Autodesk Fusion 360 part; units mm, degrees
(part 5 of 6)
sketch "b left  projection" plane through (0, 0, 0) normal (0, 0, 1) x (1, 0, 0) in component "b left component"
  arc A0 (116.825, 236.4194) -> (116.825, 235.2313) centre (117.6356, 235.8254) ccw
  arc A1 (118.4308, 236.44) -> (116.8405, 236.44) centre (117.6356, 235.8254) ccw
  arc A2 (105.08, 252.4508) -> (105.08, 250.8605) centre (105.6946, 251.6556) ccw
  arc A3 (116.8405, 226.6) -> (118.4308, 226.6) centre (117.6356, 227.2146) ccw
  arc A4 (93.7113, 250.845) -> (94.8994, 250.845) centre (94.3054, 251.6556) ccw
  arc A5 (116.825, 216.4194) -> (116.825, 215.2313) centre (117.6356, 215.8254) ccw
  arc A6 (85.08, 252.4508) -> (85.08, 250.8605) centre (85.6946, 251.6556) ccw
  arc A7 (116.8405, 206.6) -> (118.4308, 206.6) centre (117.6356, 207.2146) ccw
  arc A8 (73.7113, 250.845) -> (74.8994, 250.845) centre (74.3054, 251.6556) ccw
  arc A9 (105.08, 192.1795) -> (105.08, 190.5892) centre (105.6946, 191.3844) ccw
  arc A10 (65.08, 252.4508) -> (65.08, 250.8605) centre (65.6946, 251.6556) ccw
  arc A11 (94.8994, 192.195) -> (93.7113, 192.195) centre (94.3054, 191.3844) ccw
  arc A12 (53.7113, 250.845) -> (54.8994, 250.845) centre (54.3054, 251.6556) ccw
  arc A13 (85.08, 192.1795) -> (85.08, 190.5892) centre (85.6946, 191.3844) ccw
  arc A14 (45.08, 252.4508) -> (45.08, 250.8605) centre (45.6946, 251.6556) ccw
  arc A15 (74.8994, 192.195) -> (73.7113, 192.195) centre (74.3054, 191.3844) ccw
  arc A16 (33.7113, 250.845) -> (34.8994, 250.845) centre (34.3054, 251.6556) ccw
  arc A17 (65.08, 192.1795) -> (65.08, 190.5892) centre (65.6946, 191.3844) ccw
  arc A18 (25.08, 252.4508) -> (25.08, 250.8605) centre (25.6946, 251.6556) ccw
  arc A19 (54.8994, 192.195) -> (53.7113, 192.195) centre (54.3054, 191.3844) ccw
  arc A20 (13.7113, 250.845) -> (14.8994, 250.845) centre (14.3054, 251.6556) ccw
  arc A21 (45.08, 192.1795) -> (45.08, 190.5892) centre (45.6946, 191.3844) ccw
  arc A22 (3.175, 235.2313) -> (3.175, 236.4194) centre (2.3644, 235.8254) ccw
  arc A23 (34.8994, 192.195) -> (33.7113, 192.195) centre (34.3054, 191.3844) ccw
  arc A24 (1.5692, 226.6) -> (3.1595, 226.6) centre (2.3644, 227.2146) ccw
  arc A25 (25.08, 192.1795) -> (25.08, 190.5892) centre (25.6946, 191.3844) ccw
  arc A26 (3.175, 215.2313) -> (3.175, 216.4194) centre (2.3644, 215.8254) ccw
  arc A27 (1.5692, 206.6) -> (3.1595, 206.6) centre (2.3644, 207.2146) ccw
  arc A28 (14.8994, 192.195) -> (13.7113, 192.195) centre (14.3054, 191.3844) ccw
  arc A29 (66.2887, 192.195) -> (65.1006, 192.195) centre (65.6946, 191.3844) ccw
  arc A30 (94.92, 250.8605) -> (94.92, 252.4508) centre (94.3054, 251.6556) ccw
  arc A31 (105.1006, 250.845) -> (106.2887, 250.845) centre (105.6946, 251.6556) ccw
  arc A32 (3.175, 206.6206) -> (3.175, 207.8087) centre (2.3644, 207.2146) ccw
  arc A33 (3.1595, 216.44) -> (1.5692, 216.44) centre (2.3644, 215.8254) ccw
  arc A34 (3.175, 226.6206) -> (3.175, 227.8087) centre (2.3644, 227.2146) ccw
  arc A35 (3.1595, 236.44) -> (1.5692, 236.44) centre (2.3644, 235.8254) ccw
  arc A36 (118.4308, 216.44) -> (116.8405, 216.44) centre (117.6356, 215.8254) ccw
  arc A37 (54.92, 190.5892) -> (54.92, 192.1795) centre (54.3054, 191.3844) ccw
  arc A38 (86.2887, 192.195) -> (85.1006, 192.195) centre (85.6946, 191.3844) ccw
  arc A39 (74.92, 190.5892) -> (74.92, 192.1795) centre (74.3054, 191.3844) ccw
  arc A40 (106.2887, 192.195) -> (105.1006, 192.195) centre (105.6946, 191.3844) ccw
  arc A41 (54.92, 250.8605) -> (54.92, 252.4508) centre (54.3054, 251.6556) ccw
  arc A42 (65.1006, 250.845) -> (66.2887, 250.845) centre (65.6946, 251.6556) ccw
  arc A43 (85.1006, 250.845) -> (86.2887, 250.845) centre (85.6946, 251.6556) ccw
  arc A44 (14.92, 250.8605) -> (14.92, 252.4508) centre (14.3054, 251.6556) ccw
  arc A45 (14.92, 190.5892) -> (14.92, 192.1795) centre (14.3054, 191.3844) ccw
  arc A46 (34.92, 190.5892) -> (34.92, 192.1795) centre (34.3054, 191.3844) ccw
  arc A47 (25.1006, 250.845) -> (26.2887, 250.845) centre (25.6946, 251.6556) ccw
  arc A48 (116.825, 207.8087) -> (116.825, 206.6206) centre (117.6356, 207.2146) ccw
  arc A49 (46.2887, 192.195) -> (45.1006, 192.195) centre (45.6946, 191.3844) ccw
  arc A50 (34.92, 250.8605) -> (34.92, 252.4508) centre (34.3054, 251.6556) ccw
  arc A51 (94.92, 190.5892) -> (94.92, 192.1795) centre (94.3054, 191.3844) ccw
  arc A52 (26.2887, 192.195) -> (25.1006, 192.195) centre (25.6946, 191.3844) ccw
  arc A53 (116.825, 227.8087) -> (116.825, 226.6206) centre (117.6356, 227.2146) ccw
  arc A54 (74.92, 250.8605) -> (74.92, 252.4508) centre (74.3054, 251.6556) ccw
  arc A55 (45.1006, 250.845) -> (46.2887, 250.845) centre (45.6946, 251.6556) ccw
  line L0 (116.825, 236.44) -> (116.8405, 236.44)
  line L1 (105.08, 250.845) -> (105.1006, 250.845)
  line L2 (106.2887, 250.845) -> (120, 250.845)
  line L3 (116.825, 226.6) -> (116.825, 226.6206)
  line L4 (116.825, 227.8087) -> (116.825, 235.2313)
  line L5 (116.825, 236.4194) -> (116.825, 236.44)
  line L6 (105.08, 254.02) -> (105.08, 252.4508)
  line L7 (105.08, 250.8605) -> (105.08, 250.845)
  line L8 (120, 226.6) -> (118.4308, 226.6)
  line L9 (116.8405, 226.6) -> (116.825, 226.6)
  line L10 (94.92, 250.845) -> (94.92, 250.8605)
  line L11 (94.92, 252.4508) -> (94.92, 254.02)
  line L12 (116.825, 216.44) -> (116.8405, 216.44)
  line L13 (118.4308, 216.44) -> (120, 216.44)
  line L14 (85.08, 250.845) -> (85.1006, 250.845)
  line L15 (86.2887, 250.845) -> (93.7113, 250.845)
  line L16 (94.8994, 250.845) -> (94.92, 250.845)
  line L17 (85.08, 254.02) -> (85.08, 252.4508)
  line L18 (85.08, 250.8605) -> (85.08, 250.845)
  line L19 (116.825, 206.6) -> (116.825, 206.6206)
  line L20 (116.825, 207.8087) -> (116.825, 215.2313)
  line L21 (116.825, 216.4194) -> (116.825, 216.44)
  line L22 (120, 206.6) -> (118.4308, 206.6)
  line L23 (116.8405, 206.6) -> (116.825, 206.6)
  line L24 (74.92, 250.845) -> (74.92, 250.8605)
  line L25 (74.92, 252.4508) -> (74.92, 254.02)
  line L26 (105.08, 192.195) -> (105.1006, 192.195)
  line L27 (106.2887, 192.195) -> (120, 192.195)
  line L28 (65.08, 250.845) -> (65.1006, 250.845)
  line L29 (66.2887, 250.845) -> (73.7113, 250.845)
  line L30 (74.8994, 250.845) -> (74.92, 250.845)
  line L31 (105.08, 189.02) -> (105.08, 190.5892)
  line L32 (105.08, 192.1795) -> (105.08, 192.195)
  line L33 (65.08, 254.02) -> (65.08, 252.4508)
  line L34 (65.08, 250.8605) -> (65.08, 250.845)
  line L35 (94.92, 192.195) -> (94.92, 192.1795)
  line L36 (94.92, 190.5892) -> (94.92, 189.02)
  line L37 (54.92, 250.845) -> (54.92, 250.8605)
  line L38 (54.92, 252.4508) -> (54.92, 254.02)
  line L39 (85.08, 192.195) -> (85.1006, 192.195)
  line L40 (86.2887, 192.195) -> (93.7113, 192.195)
  line L41 (94.8994, 192.195) -> (94.92, 192.195)
  line L42 (45.08, 250.845) -> (45.1006, 250.845)
  line L43 (46.2887, 250.845) -> (53.7113, 250.845)
  line L44 (54.8994, 250.845) -> (54.92, 250.845)
  line L45 (85.08, 189.02) -> (85.08, 190.5892)
  line L46 (85.08, 192.1795) -> (85.08, 192.195)
  line L47 (45.08, 254.02) -> (45.08, 252.4508)
  line L48 (45.08, 250.8605) -> (45.08, 250.845)
  line L49 (74.92, 192.195) -> (74.92, 192.1795)
  line L50 (74.92, 190.5892) -> (74.92, 189.02)
  line L51 (34.92, 250.845) -> (34.92, 250.8605)
  line L52 (34.92, 252.4508) -> (34.92, 254.02)
  line L53 (65.08, 192.195) -> (65.1006, 192.195)
  line L54 (66.2887, 192.195) -> (73.7113, 192.195)
  line L55 (74.8994, 192.195) -> (74.92, 192.195)
  line L56 (25.08, 250.845) -> (25.1006, 250.845)
  line L57 (26.2887, 250.845) -> (33.7113, 250.845)
  line L58 (34.8994, 250.845) -> (34.92, 250.845)
  line L59 (65.08, 189.02) -> (65.08, 190.5892)
  line L60 (65.08, 192.1795) -> (65.08, 192.195)
  line L61 (25.08, 254.02) -> (25.08, 252.4508)
  line L62 (25.08, 250.8605) -> (25.08, 250.845)
  line L63 (54.92, 192.195) -> (54.92, 192.1795)
  line L64 (54.92, 190.5892) -> (54.92, 189.02)
  line L65 (14.92, 250.845) -> (14.92, 250.8605)
  line L66 (14.92, 252.4508) -> (14.92, 254.02)
  line L67 (0, 250.845) -> (13.7113, 250.845)
  line L68 (14.8994, 250.845) -> (14.92, 250.845)
  line L69 (45.08, 192.195) -> (45.1006, 192.195)
  line L70 (46.2887, 192.195) -> (53.7113, 192.195)
  line L71 (54.8994, 192.195) -> (54.92, 192.195)
  line L72 (3.175, 236.44) -> (3.1595, 236.44)
  line L73 (1.5692, 236.44) -> (0, 236.44)
  line L74 (45.08, 189.02) -> (45.08, 190.5892)
  line L75 (45.08, 192.1795) -> (45.08, 192.195)
  line L76 (34.92, 192.195) -> (34.92, 192.1795)
  line L77 (34.92, 190.5892) -> (34.92, 189.02)
  line L78 (3.175, 226.6) -> (3.175, 226.6206)
  line L79 (3.175, 227.8087) -> (3.175, 235.2313)
  line L80 (3.175, 236.4194) -> (3.175, 236.44)
  line L81 (0, 226.6) -> (1.5692, 226.6)
  line L82 (3.1595, 226.6) -> (3.175, 226.6)
  line L83 (25.08, 192.195) -> (25.1006, 192.195)
  line L84 (26.2887, 192.195) -> (33.7113, 192.195)
  line L85 (34.8994, 192.195) -> (34.92, 192.195)
  line L86 (3.175, 216.44) -> (3.1595, 216.44)
  line L87 (1.5692, 216.44) -> (0, 216.44)
  line L88 (25.08, 189.02) -> (25.08, 190.5892)
  line L89 (25.08, 192.1795) -> (25.08, 192.195)
  line L90 (3.175, 206.6) -> (3.175, 206.6206)
  line L91 (3.175, 207.8087) -> (3.175, 215.2313)
  line L92 (3.175, 216.4194) -> (3.175, 216.44)
  line L93 (14.92, 192.195) -> (14.92, 192.1795)
  line L94 (14.92, 190.5892) -> (14.92, 189.02)
  line L95 (0, 206.6) -> (1.5692, 206.6)
  line L96 (3.1595, 206.6) -> (3.175, 206.6)
  line L97 (120, 216.44) -> (120, 226.6)
  line L98 (120, 192.195) -> (120, 206.6)
  line L99 (94.92, 189.02) -> (105.08, 189.02)
  line L100 (74.92, 189.02) -> (85.08, 189.02)
  line L101 (54.92, 189.02) -> (65.08, 189.02)
  line L102 (34.92, 189.02) -> (45.08, 189.02)
  line L103 (14.92, 189.02) -> (25.08, 189.02)
  line L104 (14.8994, 192.195) -> (14.92, 192.195)
  line L105 (0, 192.195) -> (13.7113, 192.195)
  line L106 (0, 192.195) -> (0, 206.6)
  line L107 (0, 216.44) -> (0, 226.6)
  line L108 (0, 236.44) -> (0, 250.845)
  line L109 (14.92, 254.02) -> (25.08, 254.02)
  line L110 (34.92, 254.02) -> (45.08, 254.02)
  line L111 (54.92, 254.02) -> (65.08, 254.02)
  line L112 (74.92, 254.02) -> (85.08, 254.02)
  line L113 (94.92, 254.02) -> (105.08, 254.02)
  line L114 (120, 236.44) -> (120, 250.845)
  line L115 (118.4308, 236.44) -> (120, 236.44)
sketch "b right lines" plane through (0, 0, 0) normal (0, 0, 1) x (1, 0, 0) in component "b right component"
  line L0 (122.01, 192.195) -> (136.93, 192.195)
  line L1 (136.93, 192.195) -> (136.93, 189.02)
  line L2 (136.93, 189.02) -> (147.09, 189.02)
  line L3 (147.09, 189.02) -> (147.09, 192.195)
  line L4 (147.09, 192.195) -> (156.93, 192.195)
  line L5 (156.93, 192.195) -> (156.93, 189.02)
  line L6 (156.93, 189.02) -> (167.09, 189.02)
  line L7 (167.09, 189.02) -> (167.09, 192.195)
  line L8 (167.09, 192.195) -> (176.93, 192.195)
  line L9 (176.93, 192.195) -> (176.93, 189.02)
  line L10 (176.93, 189.02) -> (187.09, 189.02)
  line L11 (187.09, 189.02) -> (187.09, 192.195)
  line L12 (187.09, 192.195) -> (196.93, 192.195)
  line L13 (196.93, 192.195) -> (196.93, 189.02)
  line L14 (196.93, 189.02) -> (207.09, 189.02)
  line L15 (207.09, 189.02) -> (207.09, 192.195)
  line L16 (207.09, 192.195) -> (216.93, 192.195)
  line L17 (216.93, 192.195) -> (216.93, 189.02)
  line L18 (216.93, 189.02) -> (227.09, 189.02)
  line L19 (227.09, 189.02) -> (227.09, 192.195)
  line L20 (227.09, 192.195) -> (242.01, 192.195)
  line L21 (242.01, 192.195) -> (242.01, 206.6)
  line L22 (242.01, 206.6) -> (238.835, 206.6)
  line L23 (238.835, 206.6) -> (238.835, 216.44)
  line L24 (238.835, 216.44) -> (242.01, 216.44)
  line L25 (242.01, 216.44) -> (242.01, 226.6)
  line L26 (242.01, 226.6) -> (238.835, 226.6)
  line L27 (238.835, 226.6) -> (238.835, 236.44)
  line L28 (238.835, 236.44) -> (242.01, 236.44)
  line L29 (242.01, 236.44) -> (242.01, 250.845)
  line L30 (122.01, 250.845) -> (136.93, 250.845)
  line L31 (136.93, 250.845) -> (136.93, 254.02)
  line L32 (136.93, 254.02) -> (147.09, 254.02)
  line L33 (147.09, 254.02) -> (147.09, 250.845)
  line L34 (147.09, 250.845) -> (156.93, 250.845)
  line L35 (156.93, 250.845) -> (156.93, 254.02)
  line L36 (156.93, 254.02) -> (167.09, 254.02)
  line L37 (167.09, 254.02) -> (167.09, 250.845)
  line L38 (167.09, 250.845) -> (176.93, 250.845)
  line L39 (176.93, 250.845) -> (176.93, 254.02)
  line L40 (176.93, 254.02) -> (187.09, 254.02)
  line L41 (187.09, 254.02) -> (187.09, 250.845)
  line L42 (187.09, 250.845) -> (196.93, 250.845)
  line L43 (196.93, 250.845) -> (196.93, 254.02)
  line L44 (196.93, 254.02) -> (207.09, 254.02)
  line L45 (207.09, 254.02) -> (207.09, 250.845)
  line L46 (207.09, 250.845) -> (216.93, 250.845)
  line L47 (216.93, 250.845) -> (216.93, 254.02)
  line L48 (216.93, 254.02) -> (227.09, 254.02)
  line L49 (227.09, 254.02) -> (227.09, 250.845)
  line L50 (227.09, 250.845) -> (242.01, 250.845)
  line L51 (122.01, 192.195) -> (122.01, 206.6)
  line L52 (122.01, 206.6) -> (125.185, 206.6)
  line L53 (125.185, 206.6) -> (125.185, 216.44)
  line L54 (125.185, 216.44) -> (122.01, 216.44)
  line L55 (122.01, 216.44) -> (122.01, 226.6)
  line L56 (122.01, 226.6) -> (125.185, 226.6)
  line L57 (125.185, 226.6) -> (125.185, 236.44)
  line L58 (125.185, 236.44) -> (122.01, 236.44)
  line L59 (122.01, 236.44) -> (122.01, 250.845)
  dimension "d5818" = 14.92
  dimension "d5819" = 3.175
  dimension "d5820" = 10.16
  dimension "d5821" = 3.175
  dimension "d5822" = 9.84
  dimension "d5823" = 3.175
  dimension "d5824" = 10.16
  dimension "d5825" = 3.175
  dimension "d5826" = 9.84
  dimension "d5827" = 3.175
  dimension "d5828" = 10.16
  dimension "d5829" = 3.175
  dimension "d5830" = 9.84
  dimension "d5831" = 3.175
  dimension "d5832" = 10.16
  dimension "d5833" = 3.175
  dimension "d5834" = 9.84
  dimension "d5835" = 3.175
  dimension "d5836" = 10.16
  dimension "d5837" = 3.175
  dimension "d5838" = 14.92
  dimension "d5849" = 14.405
  dimension "d5850" = 3.175
  dimension "d5851" = 9.84
  dimension "d5852" = 3.175
  dimension "d5853" = 10.16
  dimension "d5854" = 3.175
  dimension "d5855" = 9.84
  dimension "d5856" = 3.175
  dimension "d5857" = 14.405
  dimension "d5862" = 14.92
  dimension "d5863" = 3.175
  dimension "d5864" = 10.16
  dimension "d5865" = 3.175
  dimension "d5866" = 9.84
  dimension "d5867" = 3.175
  dimension "d5868" = 10.16
  dimension "d5869" = 3.175
  dimension "d5870" = 9.84
  dimension "d5871" = 3.175
  dimension "d5872" = 10.16
  dimension "d5873" = 3.175
  dimension "d5874" = 9.84
  dimension "d5875" = 3.175
  dimension "d5876" = 10.16
  dimension "d5877" = 3.175
  dimension "d5878" = 9.84
  dimension "d5879" = 3.175
  dimension "d5880" = 10.16
  dimension "d5881" = 3.175
  dimension "d5882" = 14.92
  dimension "d5893" = 14.405
  dimension "d5894" = 3.175
  dimension "d5895" = 9.84
  dimension "d5896" = 3.175
  dimension "d5897" = 10.16
  dimension "d5898" = 3.175
  dimension "d5899" = 9.84
  dimension "d5900" = 3.175
  dimension "d5901" = 14.405
  constraint horizontal L0
  constraint vertical L1
  constraint horizontal L2
  constraint vertical L3
  constraint horizontal L4
  constraint vertical L5
  constraint horizontal L6
  constraint vertical L7
  constraint horizontal L8
  constraint vertical L9
  constraint horizontal L10
  constraint vertical L11
  constraint horizontal L12
  constraint vertical L13
  constraint horizontal L14
  constraint vertical L15
  constraint horizontal L16
  constraint vertical L17
  constraint horizontal L18
  constraint vertical L19
  constraint horizontal L20
  constraint vertical L21
  constraint horizontal L22
  constraint vertical L23
  constraint horizontal L24
  constraint vertical L25
  constraint horizontal L26
  constraint vertical L27
  constraint horizontal L28
  constraint vertical L29
  constraint horizontal L30
  constraint vertical L31
  constraint horizontal L32
  constraint vertical L33
  constraint horizontal L34
  constraint vertical L35
  constraint horizontal L36
  constraint vertical L37
  constraint horizontal L38
  constraint vertical L39
  constraint horizontal L40
  constraint vertical L41
  constraint horizontal L42
  constraint vertical L43
  constraint horizontal L44
  constraint vertical L45
  constraint horizontal L46
  constraint vertical L47
  constraint horizontal L48
  constraint vertical L49
  constraint horizontal L50
  constraint vertical L51
  constraint horizontal L52
  constraint vertical L53
  constraint horizontal L54
  constraint vertical L55
  constraint horizontal L56
  constraint vertical L57
  constraint horizontal L58
  constraint vertical L59
  measures "d5818" distance of L0.start L0.end
  measures "d5819" distance of L0.end L1.end
  measures "d5820" distance of L1.end L2.end
  measures "d5821" distance of L2.end L3.end
  measures "d5822" distance of L3.end L4.end
  measures "d5823" distance of L4.end L5.end
  measures "d5824" distance of L5.end L6.end
  measures "d5825" distance of L6.end L7.end
  measures "d5826" distance of L7.end L8.end
  measures "d5827" distance of L8.end L9.end
  measures "d5828" distance of L9.end L10.end
  measures "d5829" distance of L10.end L11.end
  measures "d5830" distance of L11.end L12.end
  measures "d5831" distance of L12.end L13.end
  measures "d5832" distance of L13.end L14.end
  measures "d5833" distance of L14.end L15.end
  measures "d5834" distance of L15.end L16.end
  measures "d5835" distance of L16.end L17.end
  measures "d5836" distance of L17.end L18.end
  measures "d5837" distance of L18.end L19.end
  measures "d5838" distance of L19.end L20.end
  measures "d5849" distance of L20.end L21.end
  measures "d5850" distance of L21.end L22.end
  measures "d5851" distance of L22.end L23.end
  measures "d5852" distance of L23.end L24.end
  measures "d5853" distance of L24.end L25.end
  measures "d5854" distance of L25.end L26.end
  measures "d5855" distance of L26.end L27.end
  measures "d5856" distance of L27.end L28.end
  measures "d5857" distance of L28.end L29.end
  measures "d5862" distance of L30.start L30.end
  measures "d5863" distance of L30.end L31.end
  measures "d5864" distance of L31.end L32.end
  measures "d5865" distance of L32.end L33.end
  measures "d5866" distance of L33.end L34.end
  measures "d5867" distance of L34.end L35.end
  measures "d5868" distance of L35.end L36.end
  measures "d5869" distance of L36.end L37.end
  measures "d5870" distance of L37.end L38.end
  measures "d5871" distance of L38.end L39.end
  measures "d5872" distance of L39.end L40.end
  measures "d5873" distance of L40.end L41.end
  measures "d5874" distance of L41.end L42.end
  measures "d5875" distance of L42.end L43.end
  measures "d5876" distance of L43.end L44.end
  measures "d5877" distance of L44.end L45.end
  measures "d5878" distance of L45.end L46.end
  measures "d5879" distance of L46.end L47.end
  measures "d5880" distance of L47.end L48.end
  measures "d5881" distance of L48.end L49.end
  measures "d5882" distance of L29.end L49.end
  measures "d5893" distance of L0.start L51.end
  measures "d5894" distance of L51.end L52.end
  measures "d5895" distance of L52.end L53.end
  measures "d5896" distance of L53.end L54.end
  measures "d5897" distance of L54.end L55.end
  measures "d5898" distance of L55.end L56.end
  measures "d5899" distance of L56.end L57.end
  measures "d5900" distance of L57.end L58.end
  measures "d5901" distance of L30.start L58.end
sketch "b right circles" plane through (0, 0, 0) normal (0, 0, 1) x (1, 0, 0) in component "b right component"
  line L0 (122.01, 189.02) -> (242.01, 189.02)
  line L1 (242.01, 189.02) -> (242.01, 254.02)
  line L2 (242.01, 254.02) -> (122.01, 254.02)
  line L3 (122.01, 254.02) -> (122.01, 189.02)
  circle A0 centre (136.3154, 191.3844) radius 1.005
  circle A1 centre (147.7046, 191.3844) radius 1.005
  circle A2 centre (156.3154, 191.3844) radius 1.005
  circle A3 centre (167.7046, 191.3844) radius 1.005
  circle A4 centre (176.3154, 191.3844) radius 1.005
  circle A5 centre (187.7046, 191.3844) radius 1.005
  circle A6 centre (196.3154, 191.3844) radius 1.005
  circle A7 centre (207.7046, 191.3844) radius 1.005
  circle A8 centre (216.3154, 191.3844) radius 1.005
  circle A9 centre (227.7046, 191.3844) radius 1.005
  circle A10 centre (239.6456, 207.2146) radius 1.005
  circle A11 centre (239.6456, 215.8254) radius 1.005
  circle A12 centre (239.6456, 227.2146) radius 1.005
  circle A13 centre (239.6456, 235.8254) radius 1.005
  circle A14 centre (136.3154, 251.6556) radius 1.005
  circle A15 centre (147.7046, 251.6556) radius 1.005
  circle A16 centre (156.3154, 251.6556) radius 1.005
  circle A17 centre (167.7046, 251.6556) radius 1.005
  circle A18 centre (176.3154, 251.6556) radius 1.005
  circle A19 centre (187.7046, 251.6556) radius 1.005
  circle A20 centre (196.3154, 251.6556) radius 1.005
  circle A21 centre (207.7046, 251.6556) radius 1.005
  circle A22 centre (216.3154, 251.6556) radius 1.005
  circle A23 centre (227.7046, 251.6556) radius 1.005
  circle A24 centre (124.3744, 207.2146) radius 1.005
  circle A25 centre (124.3744, 215.8254) radius 1.005
  circle A26 centre (124.3744, 227.2146) radius 1.005
  circle A27 centre (124.3744, 235.8254) radius 1.005
  dimension "d5839" = 2.01
  dimension "d5840" = 2.01
  dimension "d5841" = 2.01
  dimension "d5842" = 2.01
  dimension "d5843" = 2.01
  dimension "d5844" = 2.01
  dimension "d5845" = 2.01
  dimension "d5846" = 2.01
  dimension "d5847" = 2.01
  dimension "d5848" = 2.01
  dimension "d5858" = 2.01
  dimension "d5859" = 2.01
  dimension "d5860" = 2.01
  dimension "d5861" = 2.01
  dimension "d5883" = 2.01
  dimension "d5884" = 2.01
  dimension "d5885" = 2.01
  dimension "d5886" = 2.01
  dimension "d5887" = 2.01
  dimension "d5888" = 2.01
  dimension "d5889" = 2.01
  dimension "d5890" = 2.01
  dimension "d5891" = 2.01
  dimension "d5892" = 2.01
  dimension "d5902" = 2.01
  dimension "d5903" = 2.01
  dimension "d5904" = 2.01
  dimension "d5905" = 2.01
  measures "d5839" diameter of A0
  measures "d5840" diameter of A1
  measures "d5841" diameter of A2
  measures "d5842" diameter of A3
  measures "d5843" diameter of A4
  measures "d5844" diameter of A5
  measures "d5845" diameter of A6
  measures "d5846" diameter of A7
  measures "d5847" diameter of A8
  measures "d5848" diameter of A9
  measures "d5858" diameter of A10
  measures "d5859" diameter of A11
  measures "d5860" diameter of A12
  measures "d5861" diameter of A13
  measures "d5883" diameter of A14
  measures "d5884" diameter of A15
  measures "d5885" diameter of A16
  measures "d5886" diameter of A17
  measures "d5887" diameter of A18
  measures "d5888" diameter of A19
  measures "d5889" diameter of A20
  measures "d5890" diameter of A21
  measures "d5891" diameter of A22
  measures "d5892" diameter of A23
  measures "d5902" diameter of A24
  measures "d5903" diameter of A25
  measures "d5904" diameter of A26
  measures "d5905" diameter of A27
extrude "b right lines body extrude" add sketch "b right lines" along normal blind 3.175 separate body makes body 12 in component "b right component"
extrude "b right circles extrude" add sketch "b right circles" along normal blind 3.175 separate body makes body 13 in component "b right component"
combine "b right lines final combine feature" operation intersect target body 12 tool bodies 13 in component "b right component"
sketch "anchors" plane through (0, 0, 0) normal (0, 0, 1) x (1, 0, 0)
  circle A0 centre (240.5499, 211.7941) radius 1.005
  circle A1 centre (300, 21) radius 1.005
  dimension "d5912" = 2.01
  dimension "d5913" = 2.01
  measures "d5912" diameter of A0
  measures "d5913" diameter of A1
sketch "b right projection" plane through (0, 0, 0) normal (0, 0, 1) x (1, 0, 0) in component "b right component"
  arc A0 (238.835, 236.4194) -> (238.835, 235.2313) centre (239.6456, 235.8254) ccw
  arc A1 (240.4408, 236.44) -> (238.8505, 236.44) centre (239.6456, 235.8254) ccw
  arc A2 (227.09, 252.4508) -> (227.09, 250.8605) centre (227.7046, 251.6556) ccw
  arc A3 (238.8505, 226.6) -> (240.4408, 226.6) centre (239.6456, 227.2146) ccw
  arc A4 (215.7213, 250.845) -> (216.9094, 250.845) centre (216.3154, 251.6556) ccw
  arc A5 (238.835, 216.4194) -> (238.835, 215.2313) centre (239.6456, 215.8254) ccw
  arc A6 (207.09, 252.4508) -> (207.09, 250.8605) centre (207.7046, 251.6556) ccw
  arc A7 (238.8505, 206.6) -> (240.4408, 206.6) centre (239.6456, 207.2146) ccw
  arc A8 (195.7213, 250.845) -> (196.9094, 250.845) centre (196.3154, 251.6556) ccw
  arc A9 (227.09, 192.1795) -> (227.09, 190.5892) centre (227.7046, 191.3844) ccw
  arc A10 (187.09, 252.4508) -> (187.09, 250.8605) centre (187.7046, 251.6556) ccw
  arc A11 (216.9094, 192.195) -> (215.7213, 192.195) centre (216.3154, 191.3844) ccw
  arc A12 (175.7213, 250.845) -> (176.9094, 250.845) centre (176.3154, 251.6556) ccw
  arc A13 (207.09, 192.1795) -> (207.09, 190.5892) centre (207.7046, 191.3844) ccw
  arc A14 (167.09, 252.4508) -> (167.09, 250.8605) centre (167.7046, 251.6556) ccw
  arc A15 (196.9094, 192.195) -> (195.7213, 192.195) centre (196.3154, 191.3844) ccw
  arc A16 (155.7213, 250.845) -> (156.9094, 250.845) centre (156.3154, 251.6556) ccw
  arc A17 (187.09, 192.1795) -> (187.09, 190.5892) centre (187.7046, 191.3844) ccw
  arc A18 (147.09, 252.4508) -> (147.09, 250.8605) centre (147.7046, 251.6556) ccw
  arc A19 (176.9094, 192.195) -> (175.7213, 192.195) centre (176.3154, 191.3844) ccw
  arc A20 (135.7213, 250.845) -> (136.9094, 250.845) centre (136.3154, 251.6556) ccw
  arc A21 (167.09, 192.1795) -> (167.09, 190.5892) centre (167.7046, 191.3844) ccw
  arc A22 (125.185, 235.2313) -> (125.185, 236.4194) centre (124.3744, 235.8254) ccw
  arc A23 (156.9094, 192.195) -> (155.7213, 192.195) centre (156.3154, 191.3844) ccw
  arc A24 (123.5792, 226.6) -> (125.1695, 226.6) centre (124.3744, 227.2146) ccw
  arc A25 (147.09, 192.1795) -> (147.09, 190.5892) centre (147.7046, 191.3844) ccw
  arc A26 (125.185, 215.2313) -> (125.185, 216.4194) centre (124.3744, 215.8254) ccw
  arc A27 (123.5792, 206.6) -> (125.1695, 206.6) centre (124.3744, 207.2146) ccw
  arc A28 (136.9094, 192.195) -> (135.7213, 192.195) centre (136.3154, 191.3844) ccw
  arc A29 (216.93, 190.5892) -> (216.93, 192.1795) centre (216.3154, 191.3844) ccw
  arc A30 (136.93, 190.5892) -> (136.93, 192.1795) centre (136.3154, 191.3844) ccw
  arc A31 (168.2987, 192.195) -> (167.1106, 192.195) centre (167.7046, 191.3844) ccw
  arc A32 (176.93, 190.5892) -> (176.93, 192.1795) centre (176.3154, 191.3844) ccw
  arc A33 (148.2987, 192.195) -> (147.1106, 192.195) centre (147.7046, 191.3844) ccw
  arc A34 (156.93, 190.5892) -> (156.93, 192.1795) centre (156.3154, 191.3844) ccw
  arc A35 (176.93, 250.8605) -> (176.93, 252.4508) centre (176.3154, 251.6556) ccw
  arc A36 (238.835, 207.8087) -> (238.835, 206.6206) centre (239.6456, 207.2146) ccw
  arc A37 (240.4408, 216.44) -> (238.8505, 216.44) centre (239.6456, 215.8254) ccw
  arc A38 (227.1106, 250.845) -> (228.2987, 250.845) centre (227.7046, 251.6556) ccw
  arc A39 (208.2987, 192.195) -> (207.1106, 192.195) centre (207.7046, 191.3844) ccw
  arc A40 (196.93, 190.5892) -> (196.93, 192.1795) centre (196.3154, 191.3844) ccw
  arc A41 (207.1106, 250.845) -> (208.2987, 250.845) centre (207.7046, 251.6556) ccw
  arc A42 (156.93, 250.8605) -> (156.93, 252.4508) centre (156.3154, 251.6556) ccw
  arc A43 (238.835, 227.8087) -> (238.835, 226.6206) centre (239.6456, 227.2146) ccw
  arc A44 (188.2987, 192.195) -> (187.1106, 192.195) centre (187.7046, 191.3844) ccw
  arc A45 (125.1695, 216.44) -> (123.5792, 216.44) centre (124.3744, 215.8254) ccw
  arc A46 (136.93, 250.8605) -> (136.93, 252.4508) centre (136.3154, 251.6556) ccw
  arc A47 (228.2987, 192.195) -> (227.1106, 192.195) centre (227.7046, 191.3844) ccw
  arc A48 (167.1106, 250.845) -> (168.2987, 250.845) centre (167.7046, 251.6556) ccw
  arc A49 (125.185, 226.6206) -> (125.185, 227.8087) centre (124.3744, 227.2146) ccw
  arc A50 (125.185, 206.6206) -> (125.185, 207.8087) centre (124.3744, 207.2146) ccw
  arc A51 (196.93, 250.8605) -> (196.93, 252.4508) centre (196.3154, 251.6556) ccw
  arc A52 (147.1106, 250.845) -> (148.2987, 250.845) centre (147.7046, 251.6556) ccw
  arc A53 (125.1695, 236.44) -> (123.5792, 236.44) centre (124.3744, 235.8254) ccw
  arc A54 (216.93, 250.8605) -> (216.93, 252.4508) centre (216.3154, 251.6556) ccw
  arc A55 (187.1106, 250.845) -> (188.2987, 250.845) centre (187.7046, 251.6556) ccw
  line L0 (238.835, 236.44) -> (238.8505, 236.44)
  line L1 (227.09, 250.845) -> (227.1106, 250.845)
  line L2 (228.2987, 250.845) -> (242.01, 250.845)
  line L3 (238.835, 226.6) -> (238.835, 226.6206)
  line L4 (238.835, 227.8087) -> (238.835, 235.2313)
  line L5 (238.835, 236.4194) -> (238.835, 236.44)
  line L6 (227.09, 254.02) -> (227.09, 252.4508)
  line L7 (227.09, 250.8605) -> (227.09, 250.845)
  line L8 (242.01, 226.6) -> (240.4408, 226.6)
  line L9 (238.8505, 226.6) -> (238.835, 226.6)
  line L10 (216.93, 250.845) -> (216.93, 250.8605)
  line L11 (216.93, 252.4508) -> (216.93, 254.02)
  line L12 (238.835, 216.44) -> (238.8505, 216.44)
  line L13 (240.4408, 216.44) -> (242.01, 216.44)
  line L14 (207.09, 250.845) -> (207.1106, 250.845)
  line L15 (208.2987, 250.845) -> (215.7213, 250.845)
  line L16 (216.9094, 250.845) -> (216.93, 250.845)
  line L17 (207.09, 254.02) -> (207.09, 252.4508)
  line L18 (207.09, 250.8605) -> (207.09, 250.845)
  line L19 (238.835, 206.6) -> (238.835, 206.6206)
  line L20 (238.835, 207.8087) -> (238.835, 215.2313)
  line L21 (238.835, 216.4194) -> (238.835, 216.44)
  line L22 (242.01, 206.6) -> (240.4408, 206.6)
  line L23 (238.8505, 206.6) -> (238.835, 206.6)
  line L24 (196.93, 250.845) -> (196.93, 250.8605)
  line L25 (196.93, 252.4508) -> (196.93, 254.02)
  line L26 (227.09, 192.195) -> (227.1106, 192.195)
  line L27 (228.2987, 192.195) -> (242.01, 192.195)
  line L28 (187.09, 250.845) -> (187.1106, 250.845)
  line L29 (188.2987, 250.845) -> (195.7213, 250.845)
  line L30 (196.9094, 250.845) -> (196.93, 250.845)
  line L31 (227.09, 189.02) -> (227.09, 190.5892)
  line L32 (227.09, 192.1795) -> (227.09, 192.195)
  line L33 (187.09, 254.02) -> (187.09, 252.4508)
  line L34 (187.09, 250.8605) -> (187.09, 250.845)
  line L35 (216.93, 192.195) -> (216.93, 192.1795)
  line L36 (216.93, 190.5892) -> (216.93, 189.02)
  line L37 (176.93, 250.845) -> (176.93, 250.8605)
  line L38 (176.93, 252.4508) -> (176.93, 254.02)
  line L39 (207.09, 192.195) -> (207.1106, 192.195)
  line L40 (208.2987, 192.195) -> (215.7213, 192.195)
  line L41 (216.9094, 192.195) -> (216.93, 192.195)
  line L42 (167.09, 250.845) -> (167.1106, 250.845)
  line L43 (168.2987, 250.845) -> (175.7213, 250.845)
  line L44 (176.9094, 250.845) -> (176.93, 250.845)
  line L45 (207.09, 189.02) -> (207.09, 190.5892)
  line L46 (207.09, 192.1795) -> (207.09, 192.195)
  line L47 (167.09, 254.02) -> (167.09, 252.4508)
  line L48 (167.09, 250.8605) -> (167.09, 250.845)
  line L49 (196.93, 192.195) -> (196.93, 192.1795)
  line L50 (196.93, 190.5892) -> (196.93, 189.02)
  line L51 (156.93, 250.845) -> (156.93, 250.8605)
  line L52 (156.93, 252.4508) -> (156.93, 254.02)
  line L53 (187.09, 192.195) -> (187.1106, 192.195)
  line L54 (188.2987, 192.195) -> (195.7213, 192.195)
  line L55 (196.9094, 192.195) -> (196.93, 192.195)
  line L56 (147.09, 250.845) -> (147.1106, 250.845)
  line L57 (148.2987, 250.845) -> (155.7213, 250.845)
  line L58 (156.9094, 250.845) -> (156.93, 250.845)
  line L59 (187.09, 189.02) -> (187.09, 190.5892)
  line L60 (187.09, 192.1795) -> (187.09, 192.195)
  line L61 (147.09, 254.02) -> (147.09, 252.4508)
  line L62 (147.09, 250.8605) -> (147.09, 250.845)
  line L63 (176.93, 192.195) -> (176.93, 192.1795)
  line L64 (176.93, 190.5892) -> (176.93, 189.02)
  line L65 (136.93, 250.845) -> (136.93, 250.8605)
  line L66 (136.93, 252.4508) -> (136.93, 254.02)
  line L67 (122.01, 250.845) -> (135.7213, 250.845)
  line L68 (136.9094, 250.845) -> (136.93, 250.845)
  line L69 (167.09, 192.195) -> (167.1106, 192.195)
  line L70 (168.2987, 192.195) -> (175.7213, 192.195)
  line L71 (176.9094, 192.195) -> (176.93, 192.195)
  line L72 (125.185, 236.44) -> (125.1695, 236.44)
  line L73 (123.5792, 236.44) -> (122.01, 236.44)
  line L74 (167.09, 189.02) -> (167.09, 190.5892)
  line L75 (167.09, 192.1795) -> (167.09, 192.195)
  line L76 (156.93, 192.195) -> (156.93, 192.1795)
  line L77 (156.93, 190.5892) -> (156.93, 189.02)
  line L78 (125.185, 226.6) -> (125.185, 226.6206)
  line L79 (125.185, 227.8087) -> (125.185, 235.2313)
  line L80 (125.185, 236.4194) -> (125.185, 236.44)
  line L81 (122.01, 226.6) -> (123.5792, 226.6)
  line L82 (125.1695, 226.6) -> (125.185, 226.6)
  line L83 (147.09, 192.195) -> (147.1106, 192.195)
  line L84 (148.2987, 192.195) -> (155.7213, 192.195)
  line L85 (156.9094, 192.195) -> (156.93, 192.195)
  line L86 (125.185, 216.44) -> (125.1695, 216.44)
  line L87 (123.5792, 216.44) -> (122.01, 216.44)
  line L88 (147.09, 189.02) -> (147.09, 190.5892)
  line L89 (147.09, 192.1795) -> (147.09, 192.195)
  line L90 (125.185, 206.6) -> (125.185, 206.6206)
  line L91 (125.185, 207.8087) -> (125.185, 215.2313)
  line L92 (125.185, 216.4194) -> (125.185, 216.44)
  line L93 (136.93, 192.195) -> (136.93, 192.1795)
  line L94 (136.93, 190.5892) -> (136.93, 189.02)
  line L95 (122.01, 206.6) -> (123.5792, 206.6)
  line L96 (125.1695, 206.6) -> (125.185, 206.6)
  line L97 (242.01, 216.44) -> (242.01, 226.6)
  line L98 (242.01, 192.195) -> (242.01, 206.6)
  line L99 (216.93, 189.02) -> (227.09, 189.02)
  line L100 (196.93, 189.02) -> (207.09, 189.02)
  line L101 (176.93, 189.02) -> (187.09, 189.02)
  line L102 (156.93, 189.02) -> (167.09, 189.02)
  line L103 (136.93, 189.02) -> (147.09, 189.02)
  line L104 (136.9094, 192.195) -> (136.93, 192.195)
  line L105 (122.01, 192.195) -> (135.7213, 192.195)
  line L106 (122.01, 192.195) -> (122.01, 206.6)
  line L107 (122.01, 216.44) -> (122.01, 226.6)
  line L108 (122.01, 236.44) -> (122.01, 250.845)
  line L109 (136.93, 254.02) -> (147.09, 254.02)
  line L110 (156.93, 254.02) -> (167.09, 254.02)
  line L111 (176.93, 254.02) -> (187.09, 254.02)
  line L112 (196.93, 254.02) -> (207.09, 254.02)
  line L113 (216.93, 254.02) -> (227.09, 254.02)
  line L114 (242.01, 236.44) -> (242.01, 250.845)
  line L115 (240.4408, 236.44) -> (242.01, 236.44)
extrude "Extrude1" add sketch "platform content" along normal blind 3.175 separate body makes body 14 in component "platform"
component "platform" placed x (1, 0, 0) y (0, 1, 0) z (0, 0, 1) at (0, 0, 0)
component "b top component" placed x (1, 0, 0) y (0, 1, 0) z (0, 0, 1) at (0, 0, 0)
component "b bottom component" placed x (1, 0, 0) y (0, 1, 0) z (0, 0, 1) at (0, 0, 0)
component "b front component" placed x (1, 0, 0) y (0, 1, 0) z (0, 0, 1) at (0, 0, 0)
component "b back component" placed x (1, 0, 0) y (0, 1, 0) z (0, 0, 1) at (0, 0, 0)
component "b left component" placed x (1, 0, 0) y (0, 1, 0) z (0, 0, 1) at (0, 0, 0)
component "b right component" placed x (1, 0, 0) y (0, 1, 0) z (0, 0, 1) at (0, 0, 0)
equation "platformMountHoles = 3 mm"
equation "pcbMountHoles = 2 mm"
equation "d372 = b_Height"
equation "d381 = b_Length"
equation "d382 = b_Height"
equation "d2094 = ballBearingHoleDiam"
equation "d2096 = platformMountHoles"
equation "d2104 = shaftCenterToMountingHoles"
equation "d2105 = shaftCenterToMountingHoles"
equation "d2844 = b_Height"
equation "d2845 = b_Depth"
equation "b_Length = 150.00 mm" comment "Length (mm)"
equation "b_Depth = 120.00 mm" comment "Depth (mm)"
equation "b_Height = 65.00 mm" comment "Height (mm)"
equation "b_Thickness = 3.175 mm" comment "Thickness (mm)"
equation "b_Tool_diameter = 2.01 mm" comment "Tool Diameter (mm)"
equation "b_Tooth_width = 10.00 mm" comment "Target Tooth Width (mm)"
equation "b_Kerf = -0.16 mm" comment "Kerf (mm)- can be negative"
equation "b_Delta_from_bottom = -0.10 mm" comment "Additional fine adjustment of bone centers from bottom of holes(mm)- positive makes smaller bottom indents"
equation "b_Stock_x_dimension = 304.80 mm" comment "Stock X Dimension *"
equation "b_Stock_y_dimension = 609.60 mm" comment "Stock Y Dimension"
equation "b_Repeats_l_tmp = -1.00 mm" comment "temp hidden"
equation "d3674 = b_Length"
equation "d3675 = b_Depth"
equation "d3676 = pcbMountHoles"
equation "d3683 = b_Tool_diameter"
equation "d3684 = 3 * b_Thickness"
equation "d3685 = 3 * b_Thickness"
equation "d3687 = 360.0 °"
equation "d3690 = b_Length - 6 * b_Thickness"
equation "d3691 = b_Depth - 6 * b_Thickness"
equation "d3693 = b_Depth + b_Tool_diameter"
equation "d3694 = b_Length + b_Tool_diameter"
equation "d3695 = b_Depth + b_Tool_diameter"
equation "d3696 = b_Depth + b_Height + 2 * b_Tool_diameter"
equation "d3712 = b_Tool_diameter"
equation "d3726 = b_Depth"
equation "d3727 = b_Tool_diameter"
equation "d3730 = b_Height"
equation "d3731 = b_Length + b_Tool_diameter"
equation "Version_info = 0 mm" comment "1.2.0 LENGTH 150.0 DEPTH 120.0 HEIGHT 65.0 THICKNESS 3.175 TOOL_DIAMETER 2.01 TOOTH_WIDTH 10.0 KERF -0.16 DELTA_FROM_BOTTOM -0.1 STOCK_X_DIMENSION 304.8 STOCK_Y_DIMENSION 609.6 COMPONENT  REPEATS_L_TMP -1 CREATE_COMPONENTS False CREATE_BODIES 1 CREATE_EMPTY_CONTENTS False CREATE_CONSTRAINTS True CLEAR_PREVIOUSLY_GENERATED_ITEMS True JUST_CLEAR_PREVIOUSLY_GENERATED_ITEMS False CREATE_MANUFACTURING False JUST_CREATE_MANUFACTURING False DEBUG_JUST_ONE_PART False MANUAL_LAYOUT  LASER False JUST_BUILD_TEST False DEBUG True"
equation "d5191 = b_Thickness"
equation "d5193 = b_Thickness"
equation "d5195 = b_Thickness"
equation "d5197 = b_Thickness"
equation "d5199 = b_Thickness"
equation "d5201 = b_Thickness"
equation "d5203 = b_Thickness"
equation "d5205 = b_Thickness"
equation "d5207 = b_Thickness"
equation "d5209 = b_Thickness"
equation "d5211 = b_Thickness"
equation "d5213 = b_Thickness"
equation "d5215 = b_Thickness"
equation "d5217 = b_Thickness"
equation "d5219 = b_Tool_diameter"
equation "d5220 = b_Tool_diameter"
equation "d5221 = b_Tool_diameter"
equation "d5222 = b_Tool_diameter"
equation "d5223 = b_Tool_diameter"
equation "d5224 = b_Tool_diameter"
equation "d5225 = b_Tool_diameter"
equation "d5226 = b_Tool_diameter"
equation "d5227 = b_Tool_diameter"
equation "d5228 = b_Tool_diameter"
equation "d5229 = b_Tool_diameter"
equation "d5230 = b_Tool_diameter"
equation "d5231 = b_Tool_diameter"
equation "d5232 = b_Tool_diameter"
equation "d5234 = b_Thickness"
equation "d5236 = b_Thickness"
equation "d5238 = b_Thickness"
equation "d5240 = b_Thickness"
equation "d5242 = b_Thickness"
equation "d5244 = b_Thickness"
equation "d5246 = b_Thickness"
equation "d5248 = b_Thickness"
equation "d5250 = b_Thickness"
equation "d5252 = b_Thickness"
equation "d5254 = b_Tool_diameter"
equation "d5255 = b_Tool_diameter"
equation "d5256 = b_Tool_diameter"
equation "d5257 = b_Tool_diameter"
equation "d5258 = b_Tool_diameter"
equation "d5259 = b_Tool_diameter"
equation "d5260 = b_Tool_diameter"
equation "d5261 = b_Tool_diameter"
equation "d5262 = b_Tool_diameter"
equation "d5263 = b_Tool_diameter"
equation "d5265 = b_Thickness"
equation "d5267 = b_Thickness"
equation "d5269 = b_Thickness"
equation "d5271 = b_Thickness"
equation "d5273 = b_Thickness"
equation "d5275 = b_Thickness"
equation "d5277 = b_Thickness"
equation "d5279 = b_Thickness"
equation "d5281 = b_Thickness"
equation "d5283 = b_Thickness"
equation "d5285 = b_Thickness"
equation "d5287 = b_Thickness"
equation "d5289 = b_Thickness"
equation "d5291 = b_Thickness"
equation "d5293 = b_Tool_diameter"
equation "d5294 = b_Tool_diameter"
equation "d5295 = b_Tool_diameter"
equation "d5296 = b_Tool_diameter"
equation "d5297 = b_Tool_diameter"
equation "d5298 = b_Tool_diameter"
equation "d5299 = b_Tool_diameter"
equation "d5300 = b_Tool_diameter"
equation "d5301 = b_Tool_diameter"
equation "d5302 = b_Tool_diameter"
equation "d5303 = b_Tool_diameter"
equation "d5304 = b_Tool_diameter"
equation "d5305 = b_Tool_diameter"
equation "d5306 = b_Tool_diameter"
equation "d5308 = b_Thickness"
equation "d5310 = b_Thickness"
equation "d5312 = b_Thickness"
equation "d5314 = b_Thickness"
equation "d5316 = b_Thickness"
equation "d5318 = b_Thickness"
equation "d5320 = b_Thickness"
equation "d5322 = b_Thickness"
equation "d5324 = b_Thickness"
equation "d5326 = b_Thickness"
equation "d5328 = b_Tool_diameter"
equation "d5329 = b_Tool_diameter"
equation "d5330 = b_Tool_diameter"
equation "d5331 = b_Tool_diameter"
equation "d5332 = b_Tool_diameter"
equation "d5333 = b_Tool_diameter"
equation "d5334 = b_Tool_diameter"
equation "d5335 = b_Tool_diameter"
equation "d5336 = b_Tool_diameter"
equation "d5337 = b_Tool_diameter"
equation "d5343 = b_Thickness"
equation "d5345 = b_Thickness"
equation "d5347 = b_Thickness"
equation "d5349 = b_Thickness"
equation "d5351 = b_Thickness"
equation "d5353 = b_Thickness"
equation "d5355 = b_Thickness"
equation "d5357 = b_Thickness"
equation "d5359 = b_Thickness"
equation "d5361 = b_Thickness"
equation "d5363 = b_Thickness"
equation "d5365 = b_Thickness"
equation "d5367 = b_Thickness"
equation "d5369 = b_Thickness"
equation "d5371 = b_Tool_diameter"
equation "d5372 = b_Tool_diameter"
equation "d5373 = b_Tool_diameter"
equation "d5374 = b_Tool_diameter"
equation "d5375 = b_Tool_diameter"
equation "d5376 = b_Tool_diameter"
equation "d5377 = b_Tool_diameter"
equation "d5378 = b_Tool_diameter"
equation "d5379 = b_Tool_diameter"
equation "d5380 = b_Tool_diameter"
equation "d5381 = b_Tool_diameter"
equation "d5382 = b_Tool_diameter"
equation "d5383 = b_Tool_diameter"
equation "d5384 = b_Tool_diameter"
equation "d5386 = b_Thickness"
equation "d5388 = b_Thickness"
equation "d5390 = b_Thickness"
equation "d5392 = b_Thickness"
equation "d5394 = b_Thickness"
equation "d5396 = b_Thickness"
equation "d5398 = b_Thickness"
equation "d5400 = b_Thickness"
equation "d5402 = b_Thickness"
equation "d5404 = b_Thickness"
equation "d5406 = b_Tool_diameter"
equation "d5407 = b_Tool_diameter"
equation "d5408 = b_Tool_diameter"
equation "d5409 = b_Tool_diameter"
equation "d5410 = b_Tool_diameter"
equation "d5411 = b_Tool_diameter"
equation "d5412 = b_Tool_diameter"
equation "d5413 = b_Tool_diameter"
equation "d5414 = b_Tool_diameter"
equation "d5415 = b_Tool_diameter"
equation "d5417 = b_Thickness"
equation "d5419 = b_Thickness"
equation "d5421 = b_Thickness"
equation "d5423 = b_Thickness"
equation "d5425 = b_Thickness"
equation "d5427 = b_Thickness"
equation "d5429 = b_Thickness"
equation "d5431 = b_Thickness"
equation "d5433 = b_Thickness"
equation "d5435 = b_Thickness"
equation "d5437 = b_Thickness"
equation "d5439 = b_Thickness"
equation "d5441 = b_Thickness"
equation "d5443 = b_Thickness"
equation "d5445 = b_Tool_diameter"
equation "d5446 = b_Tool_diameter"
equation "d5447 = b_Tool_diameter"
equation "d5448 = b_Tool_diameter"
equation "d5449 = b_Tool_diameter"
equation "d5450 = b_Tool_diameter"
equation "d5451 = b_Tool_diameter"
equation "d5452 = b_Tool_diameter"
equation "d5453 = b_Tool_diameter"
equation "d5454 = b_Tool_diameter"
equation "d5455 = b_Tool_diameter"
equation "d5456 = b_Tool_diameter"
equation "d5457 = b_Tool_diameter"
equation "d5458 = b_Tool_diameter"
equation "d5460 = b_Thickness"
equation "d5462 = b_Thickness"
equation "d5464 = b_Thickness"
equation "d5466 = b_Thickness"
equation "d5468 = b_Thickness"
equation "d5470 = b_Thickness"
equation "d5472 = b_Thickness"
equation "d5474 = b_Thickness"
equation "d5476 = b_Thickness"
equation "d5478 = b_Thickness"
equation "d5480 = b_Tool_diameter"
equation "d5481 = b_Tool_diameter"
equation "d5482 = b_Tool_diameter"
equation "d5483 = b_Tool_diameter"
equation "d5484 = b_Tool_diameter"
equation "d5485 = b_Tool_diameter"
equation "d5486 = b_Tool_diameter"
equation "d5487 = b_Tool_diameter"
equation "d5488 = b_Tool_diameter"
equation "d5489 = b_Tool_diameter"
equation "d5495 = b_Thickness"
equation "d5497 = b_Thickness"
equation "d5499 = b_Thickness"
equation "d5501 = b_Thickness"
equation "d5503 = b_Thickness"
equation "d5505 = b_Thickness"
equation "d5507 = b_Thickness"
equation "d5509 = b_Thickness"
equation "d5511 = b_Thickness"
equation "d5513 = b_Thickness"
equation "d5515 = b_Thickness"
equation "d5517 = b_Thickness"
equation "d5519 = b_Thickness"
equation "d5521 = b_Thickness"
equation "d5523 = b_Tool_diameter"
equation "d5524 = b_Tool_diameter"
equation "d5525 = b_Tool_diameter"
equation "d5526 = b_Tool_diameter"
equation "d5527 = b_Tool_diameter"
equation "d5528 = b_Tool_diameter"
equation "d5529 = b_Tool_diameter"
equation "d5530 = b_Tool_diameter"
equation "d5531 = b_Tool_diameter"
equation "d5532 = b_Tool_diameter"
equation "d5533 = b_Tool_diameter"
equation "d5534 = b_Tool_diameter"
equation "d5535 = b_Tool_diameter"
equation "d5536 = b_Tool_diameter"
equation "d5538 = b_Thickness"
equation "d5540 = b_Thickness"
equation "d5542 = b_Thickness"
equation "d5544 = b_Thickness"
equation "d5546 = b_Tool_diameter"
equation "d5547 = b_Tool_diameter"
equation "d5548 = b_Tool_diameter"
equation "d5549 = b_Tool_diameter"
equation "d5551 = b_Thickness"
equation "d5553 = b_Thickness"
equation "d5555 = b_Thickness"
equation "d5557 = b_Thickness"
equation "d5559 = b_Thickness"
equation "d5561 = b_Thickness"
equation "d5563 = b_Thickness"
equation "d5565 = b_Thickness"
equation "d5567 = b_Thickness"
equation "d5569 = b_Thickness"
equation "d5571 = b_Thickness"
equation "d5573 = b_Thickness"
equation "d5575 = b_Thickness"
equation "d5577 = b_Thickness"
equation "d5579 = b_Tool_diameter"
equation "d5580 = b_Tool_diameter"
equation "d5581 = b_Tool_diameter"
equation "d5582 = b_Tool_diameter"
equation "d5583 = b_Tool_diameter"
equation "d5584 = b_Tool_diameter"
equation "d5585 = b_Tool_diameter"
equation "d5586 = b_Tool_diameter"
equation "d5587 = b_Tool_diameter"
equation "d5588 = b_Tool_diameter"
equation "d5589 = b_Tool_diameter"
equation "d5590 = b_Tool_diameter"
equation "d5591 = b_Tool_diameter"
equation "d5592 = b_Tool_diameter"
equation "d5594 = b_Thickness"
equation "d5596 = b_Thickness"
equation "d5598 = b_Thickness"
equation "d5600 = b_Thickness"
equation "d5602 = b_Tool_diameter"
equation "d5603 = b_Tool_diameter"
equation "d5604 = b_Tool_diameter"
equation "d5605 = b_Tool_diameter"
equation "d5611 = b_Thickness"
equation "d5613 = b_Thickness"
equation "d5615 = b_Thickness"
equation "d5617 = b_Thickness"
equation "d5619 = b_Thickness"
equation "d5621 = b_Thickness"
equation "d5623 = b_Thickness"
equation "d5625 = b_Thickness"
equation "d5627 = b_Thickness"
equation "d5629 = b_Thickness"
equation "d5631 = b_Thickness"
equation "d5633 = b_Thickness"
equation "d5635 = b_Thickness"
equation "d5637 = b_Thickness"
equation "d5639 = b_Tool_diameter"
equation "d5640 = b_Tool_diameter"
equation "d5641 = b_Tool_diameter"
equation "d5642 = b_Tool_diameter"
equation "d5643 = b_Tool_diameter"
equation "d5644 = b_Tool_diameter"
equation "d5645 = b_Tool_diameter"
equation "d5646 = b_Tool_diameter"
equation "d5647 = b_Tool_diameter"
equation "d5648 = b_Tool_diameter"
equation "d5649 = b_Tool_diameter"
equation "d5650 = b_Tool_diameter"
equation "d5651 = b_Tool_diameter"
equation "d5652 = b_Tool_diameter"
equation "d5654 = b_Thickness"
equation "d5656 = b_Thickness"
equation "d5658 = b_Thickness"
equation "d5660 = b_Thickness"
equation "d5662 = b_Tool_diameter"
equation "d5663 = b_Tool_diameter"
equation "d5664 = b_Tool_diameter"
equation "d5665 = b_Tool_diameter"
equation "d5667 = b_Thickness"
equation "d5669 = b_Thickness"
equation "d5671 = b_Thickness"
equation "d5673 = b_Thickness"
equation "d5675 = b_Thickness"
equation "d5677 = b_Thickness"
equation "d5679 = b_Thickness"
equation "d5681 = b_Thickness"
equation "d5683 = b_Thickness"
equation "d5685 = b_Thickness"
equation "d5687 = b_Thickness"
equation "d5689 = b_Thickness"
equation "d5691 = b_Thickness"
equation "d5693 = b_Thickness"
equation "d5695 = b_Tool_diameter"
equation "d5696 = b_Tool_diameter"
equation "d5697 = b_Tool_diameter"
equation "d5698 = b_Tool_diameter"
equation "d5699 = b_Tool_diameter"
equation "d5700 = b_Tool_diameter"
equation "d5701 = b_Tool_diameter"
equation "d5702 = b_Tool_diameter"
equation "d5703 = b_Tool_diameter"
equation "d5704 = b_Tool_diameter"
equation "d5705 = b_Tool_diameter"
equation "d5706 = b_Tool_diameter"
equation "d5707 = b_Tool_diameter"
equation "d5708 = b_Tool_diameter"
equation "d5710 = b_Thickness"
equation "d5712 = b_Thickness"
equation "d5714 = b_Thickness"
equation "d5716 = b_Thickness"
equation "d5718 = b_Tool_diameter"
equation "d5719 = b_Tool_diameter"
equation "d5720 = b_Tool_diameter"
equation "d5721 = b_Tool_diameter"
equation "d5727 = b_Thickness"
equation "d5729 = b_Thickness"
equation "d5731 = b_Thickness"
equation "d5733 = b_Thickness"
equation "d5735 = b_Thickness"
equation "d5737 = b_Thickness"
equation "d5739 = b_Thickness"
equation "d5741 = b_Thickness"
equation "d5743 = b_Thickness"
equation "d5745 = b_Thickness"
equation "d5747 = b_Tool_diameter"
equation "d5748 = b_Tool_diameter"
equation "d5749 = b_Tool_diameter"
equation "d5750 = b_Tool_diameter"
equation "d5751 = b_Tool_diameter"
equation "d5752 = b_Tool_diameter"
equation "d5753 = b_Tool_diameter"
equation "d5754 = b_Tool_diameter"
equation "d5755 = b_Tool_diameter"
equation "d5756 = b_Tool_diameter"
equation "d5758 = b_Thickness"
equation "d5760 = b_Thickness"
equation "d5762 = b_Thickness"
equation "d5764 = b_Thickness"
equation "d5766 = b_Tool_diameter"
equation "d5767 = b_Tool_diameter"
equation "d5768 = b_Tool_diameter"
equation "d5769 = b_Tool_diameter"
equation "d5771 = b_Thickness"
equation "d5773 = b_Thickness"
equation "d5775 = b_Thickness"
equation "d5777 = b_Thickness"
equation "d5779 = b_Thickness"
equation "d5781 = b_Thickness"
equation "d5783 = b_Thickness"
equation "d5785 = b_Thickness"
equation "d5787 = b_Thickness"
equation "d5789 = b_Thickness"
equation "d5791 = b_Tool_diameter"
equation "d5792 = b_Tool_diameter"
equation "d5793 = b_Tool_diameter"
equation "d5794 = b_Tool_diameter"